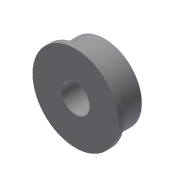
# Autodesk Inventor part: 00_ballbearing_8mm
Saved by Autodesk Inventor 2019.4 (Build 234330000, 330)
## iProperties
Created: 2021-09-13
Part Number: 00_ballbearing_8mm
Material: Generic
Document SubType Name: Modeling
Designer: diederichbenedict
Density: 1 g/cm^3
Appearance: Default
Author: diederichbenedict
Autodesk Inventor part; units mm, degrees
ref_plane "YZ Plane" through (0, 0, 0) normal (1, 0, 0) x (0, 1, 0)
ref_plane "XZ Plane" through (0, 0, 0) normal (0, 1, 0) x (-1, 0, 0)
ref_plane "XY Plane" through (0, 0, 0) normal (0, 0, 1) x (1, 0, 0)
sketch "Sketch1" plane through (0, 0, 0) normal (0, 1, 0) x (-1, 0, 0)
  line L0 (16.6772, 52.6366) -> (16.6772, 50.1366)
  line L1 (16.6772, 50.1366) -> (19.1772, 50.1366)
  line L2 (19.1772, 50.1366) -> (19.1772, 52.6421)
  line L3 (19.1772, 52.6421) -> (19.7772, 52.6421)
  line L4 (19.7772, 52.6421) -> (19.7772, 53.2421)
  line L5 (19.7772, 53.2421) -> (16.6772, 53.2421)
  line L6 (16.6772, 53.2421) -> (16.6772, 52.6366)
  line L7 (15.1772, 53.2421) -> (15.1772, 48.9703)
  point P0 (0, 0)
  dimension "d0" = 2.5
  dimension "d1" = 1.5
  dimension "d2" = 2.5
  dimension "d3" = 0.6
  dimension "d4" = 0.6
  dimension "d5" = 0
  constraints: 16 end point, 3 perpendicular, 2 parallel, 2 point on line, 1 collinear, 1 vertical
  measures "d0" distance of L0.start L0.end
  measures "d1" distance between parallel lines of L6 L7
  measures "d2" distance between parallel lines of L0 L2
  measures "d3" distance between parallel lines of L2 L4
  measures "d4" distance between parallel lines of L5 L3
  measures "d5" angle of L5 L1
revolve "Revolution1" add sketch "Sketch1" angle 360 about axis through (-15.1772, 0, 53.2421) along (0, 0, -1)
body "Solid1"
